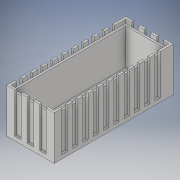
# Autodesk Inventor part: COINTAITER
Saved by Autodesk Inventor 2019 (Build 230136000, 136)
## iProperties
Created: 2020-08-23
Part Number: COINTAITER
Material: Generic
Document SubType Name: Modeling
Designer: mihai
Density: 1 g/cm^3
Appearance: Default
Author: mihai
Autodesk Inventor part; units mm, degrees
ref_plane "YZ Plane" through (0, 0, 0) normal (1, 0, 0) x (0, 1, 0)
ref_plane "XZ Plane" through (0, 0, 0) normal (0, 1, 0) x (-1, 0, 0)
ref_plane "XY Plane" through (0, 0, 0) normal (0, 0, 1) x (1, 0, 0)
sketch "Sketch1" plane through (0, 0, 0) normal (0, 1, 0) x (-1, 0, 0)
  line L0 (0, 0) -> (0, -147.45)
  line L1 (0, -147.45) -> (58.8, -147.45)
  line L2 (58.8, -147.45) -> (58.8, 0)
  line L3 (58.8, 0) -> (0, 0)
  dimension "d0" = 147.45
  dimension "d1" = 58.8
  constraints: 8 end point, 3 perpendicular, 1 vertical
  measures "d0" distance of L0.start L0.end
  measures "d1" distance of L0.end L1.end
extrude "Extrusion1" add sketch "Sketch1" along normal blind 5
sketch "Sketch2" plane through (0, 5, 0) normal (0, 1, 0) x (1, 0, 0)
  line L0 (0, 0) -> (0, 147.45) projected
  line L1 (0, 147.45) -> (-58.8, 147.45) projected
  line L2 (-58.8, 147.45) -> (-58.8, 0) projected
  line L3 (-58.8, 0) -> (0, 0) projected
  line L4 (0, 0) -> (0, 147.45) projected
  line L5 (0, 0) -> (-10, 0)
  line L6 (-10, 0) -> (-10, 5)
  line L7 (-10, 5) -> (-5, 5)
  line L8 (-5, 5) -> (-5, 10)
  line L9 (-5, 10) -> (0, 10)
  line L10 (0, 0) -> (0, 10)
  line L11 (0, 147.45) -> (0, 137.45)
  line L12 (0, 137.45) -> (-5, 137.45)
  line L13 (-5, 137.45) -> (-5, 142.45)
  line L14 (-5, 142.45) -> (-10, 142.45)
  line L15 (-10, 142.45) -> (-10, 147.45)
  line L16 (0, 147.45) -> (-58.8, 147.45) projected
  line L17 (-10, 147.45) -> (0, 147.45)
  line L18 (-58.8, 147.45) -> (-58.8, 137.45)
  line L19 (-53.8, 137.45) -> (-53.8, 142.45)
  line L20 (-53.8, 142.45) -> (-48.8, 142.45)
  line L21 (-48.8, 142.45) -> (-48.8, 147.45)
  line L22 (-48.8, 147.45) -> (-58.8, 147.45)
  line L23 (-58.8, 137.45) -> (-53.8, 137.45)
  line L24 (-58.8, 147.45) -> (-58.8, 0) projected
  line L25 (-58.8, 0) -> (-58.8, 10)
  line L26 (-58.8, 10) -> (-53.8, 10)
  line L27 (-53.8, 10) -> (-53.8, 5)
  line L28 (-53.8, 5) -> (-48.8, 5)
  line L29 (-48.8, 5) -> (-48.8, 0)
  line L30 (-58.8, 0) -> (0, 0) projected
  line L31 (-48.8, 0) -> (-58.8, 0)
  dimension "d7" = 10
  dimension "d8" = 10
  constraints: 48 end point, 13 perpendicular, 10 point on line, 2 collinear, 1 horizontal, 1 parallel, 1 vertical
  measures "d7" distance of L4.start L5.end
  measures "d8" distance of L0.end L11.end
extrude "Extrusion2" add sketch "Sketch2" along normal blind 49.575 contours L3 L6 L7 L8 L9 L0 | L12 L13 L14 L15 L1 L0 | L3 L2 L26 L27 L28 L29 | L21 L20 L19 L23 L2 L1
sketch "Sketch3" plane through (0, 5, 0) normal (0, 1, 0) x (1, 0, 0)
  line L0 (-5, 10) -> (0, 10) projected
  line L1 (-2.5, 10) -> (-2.5, 16.3725) construction
  line L2 (-2.5, 16.3725) -> (-2.5, 22.745) construction
  line L3 (-2.5, 10) -> (-2.5, 16.3725)
  line L4 (-2.5, 16.3725) -> (0, 16.3725)
  line L5 (0, 16.3725) -> (0, 22.745)
  line L6 (0, 22.745) -> (-2.5, 22.745)
  line L7 (-5, 5) -> (-5, 10) projected
  line L8 (-5, 137.45) -> (0, 137.45) projected
  line L9 (-5, 10) -> (-5, 137.45)
  line L10 (-10, 142.45) -> (-10, 147.45) projected
  line L11 (-53.8, 142.45) -> (-48.8, 142.45) projected
  line L12 (-10, 142.45) -> (-48.8, 142.45)
  line L13 (-53.8, 137.45) -> (-53.8, 10)
  line L14 (-48.8, 5) -> (-48.8, 0) projected
  line L15 (-48.8, 5) -> (-10, 5)
  line L16 (-2.5, 22.745) -> (-2.5, 29.1175)
  line L17 (-2.5, 29.1175) -> (0, 29.1175)
  line L18 (0, 29.1175) -> (0, 35.49)
  line L19 (0, 35.49) -> (-2.5, 35.49)
  line L20 (-2.5, 35.49) -> (-2.5, 41.8625)
  line L21 (-2.5, 41.8625) -> (0, 41.8625)
  line L22 (0, 41.8625) -> (0, 48.235)
  line L23 (0, 48.235) -> (-2.5, 48.235)
  line L24 (-2.5, 48.235) -> (-2.5, 54.6075)
  line L25 (-2.5, 54.6075) -> (0, 54.6075)
  line L26 (0, 54.6075) -> (0, 60.98)
  line L27 (0, 60.98) -> (-2.5, 60.98)
  line L28 (-2.5, 60.98) -> (-2.5, 67.3525)
  line L29 (-2.5, 67.3525) -> (0, 67.3525)
  line L30 (0, 67.3525) -> (0, 73.725)
  line L31 (0, 73.725) -> (-2.5, 73.725)
  line L32 (-2.5, 73.725) -> (-2.5, 80.0975)
  line L33 (-2.5, 80.0975) -> (0, 80.0975)
  line L34 (0, 80.0975) -> (0, 86.47)
  line L35 (0, 86.47) -> (-2.5, 86.47)
  line L36 (-2.5, 86.47) -> (-2.5, 92.8425)
  line L37 (-2.5, 92.8425) -> (0, 92.8425)
  line L38 (0, 92.8425) -> (0, 99.215)
  line L39 (0, 99.215) -> (-2.5, 99.215)
  line L40 (-2.5, 99.215) -> (-2.5, 105.5875)
  line L41 (-2.5, 105.5875) -> (0, 105.5875)
  line L42 (0, 105.5875) -> (0, 111.96)
  line L43 (0, 111.96) -> (-2.5, 111.96)
  line L44 (-2.5, 111.96) -> (-2.5, 118.3325)
  line L45 (-2.5, 118.3325) -> (0, 118.3325)
  line L46 (0, 118.3325) -> (0, 124.705)
  line L47 (0, 124.705) -> (-2.5, 124.705)
  line L48 (-2.5, 124.705) -> (-2.5, 131.0775)
  line L49 (-2.5, 131.0775) -> (0, 131.0775)
  line L50 (0, 131.0775) -> (0, 137.45)
  line L51 (0, 137.45) -> (-2.5, 137.45)
  line L52 (-5, 10) -> (-2.5, 10)
  line L53 (0, 10) -> (0, 137.45) projected
  line L54 (-5, 137.45) -> (0, 137.45)
  point P0 (0, 0)
  dimension "d11" = 6.3725
  dimension "d12" = 6.3725
  constraints: 96 end point, 4 horizontal, 4 vertical, 2 collinear, 1 midpoint, 1 perpendicular, 1 other
  measures "d11" distance of L1.start L1.end
  measures "d12" distance of L2.end L1.end
extrude "Extrusion3" add sketch "Sketch3" along normal blind 49.575 contours L9 L8 L50 L49 L48 L47 L46 L45 L44 L43 L42 L41 L40 L39 L38 L37 L36 L35 L34 L33 L32 L31 L30 L29 L28 L27 L26 L25 L24 L23 L22 L21 L20 L19 L18 L17 L16 L6 L5 L4 L3 L0
sketch "Sketch4" plane through (0, 5, 0) normal (0, 1, 0) x (1, 0, 0)
  line L0 (-2.5, 10) -> (-2.5, 16.3725) projected
  line L1 (0, 10) -> (-2.5, 10) projected
  line L2 (-58.8, 10) -> (-53.8, 10) projected
  line L3 (-56.3, 10) -> (-56.3, 16.3725)
  line L4 (-56.3, 16.3725) -> (-58.8, 16.3725)
  line L5 (0, 16.3725) -> (0, 22.745) projected
  line L6 (0, 22.745) -> (-2.5, 22.745) projected
  line L7 (-58.8, 16.3725) -> (-58.8, 22.745)
  line L8 (-58.8, 22.745) -> (-56.3, 22.745)
  line L9 (-5, 142.45) -> (-5, 5) projected
  line L10 (-56.3, 22.745) -> (-56.3, 29.1175)
  line L11 (-56.3, 29.1175) -> (-58.8, 29.1175)
  line L12 (-58.8, 29.1175) -> (-58.8, 35.49)
  line L13 (-58.8, 35.49) -> (-56.3, 35.49)
  line L14 (-56.3, 35.49) -> (-56.3, 41.8625)
  line L15 (-56.3, 41.8625) -> (-58.8, 41.8625)
  line L16 (-58.8, 41.8625) -> (-58.8, 48.235)
  line L17 (-58.8, 48.235) -> (-56.3, 48.235)
  line L18 (-56.3, 48.235) -> (-56.3, 54.6075)
  line L19 (-56.3, 54.6075) -> (-58.8, 54.6075)
  line L20 (-58.8, 54.6075) -> (-58.8, 60.98)
  line L21 (-58.8, 60.98) -> (-56.3, 60.98)
  line L22 (-56.3, 60.98) -> (-56.3, 67.3525)
  line L23 (-56.3, 67.3525) -> (-58.8, 67.3525)
  line L24 (-58.8, 67.3525) -> (-58.8, 73.725)
  line L25 (-58.8, 73.725) -> (-56.3, 73.725)
  line L26 (-56.3, 73.725) -> (-56.3, 80.0975)
  line L27 (-56.3, 80.0975) -> (-58.8, 80.0975)
  line L28 (-58.8, 80.0975) -> (-58.8, 86.47)
  line L29 (-58.8, 86.47) -> (-56.3, 86.47)
  line L30 (-56.3, 86.47) -> (-56.3, 92.8425)
  line L31 (-56.3, 92.8425) -> (-58.8, 92.8425)
  line L32 (-58.8, 92.8425) -> (-58.8, 99.215)
  line L33 (-58.8, 99.215) -> (-56.3, 99.215)
  line L34 (-56.3, 99.215) -> (-56.3, 105.5875)
  line L35 (-56.3, 105.5875) -> (-58.8, 105.5875)
  line L36 (-58.8, 105.5875) -> (-58.8, 111.96)
  line L37 (-58.8, 111.96) -> (-56.3, 111.96)
  line L38 (-56.3, 111.96) -> (-56.3, 118.3325)
  line L39 (-56.3, 118.3325) -> (-58.8, 118.3325)
  line L40 (-58.8, 118.3325) -> (-58.8, 124.705)
  line L41 (-58.8, 124.705) -> (-56.3, 124.705)
  line L42 (-56.3, 124.705) -> (-56.3, 131.0775)
  line L43 (-56.3, 131.0775) -> (-58.8, 131.0775)
  line L44 (-58.8, 131.0775) -> (-58.8, 137.45)
  line L45 (-58.8, 137.45) -> (-56.3, 137.45)
  line L46 (-58.8, 137.45) -> (-53.8, 137.45) projected
  line L47 (-56.3, 137.45) -> (-53.8, 137.45)
  line L48 (-53.8, 137.45) -> (-53.8, 10)
  line L49 (-56.3, 10) -> (-53.8, 10)
  point P0 (0, 0)
  constraints: 86 end point, 2 collinear, 2 perpendicular, 1 horizontal, 1 midpoint, 1 vertical
extrude "Extrusion4" add sketch "Sketch4" along normal blind 49.575
sketch "Sketch5" plane through (0, 5, 0) normal (0, 1, 0) x (1, 0, 0)
  line L0 (-10, 0) -> (-10, 5) projected
  line L1 (-10, 2.5) -> (-17.771, 2.5)
  line L2 (-17.771, 2.5) -> (-17.771, 0)
  line L3 (-17.771, 0) -> (-25.542, 0)
  line L4 (-25.542, 0) -> (-25.542, 2.5)
  line L5 (-5, 5) -> (-10, 5) projected
  line L6 (-25.542, 2.5) -> (-33.313, 2.5)
  line L7 (-33.313, 2.5) -> (-33.313, 0)
  line L8 (-33.313, 0) -> (-41.084, 0)
  line L9 (-48.8, 0) -> (-10, 0) projected
  line L10 (-41.084, 0) -> (-41.084, 2.5)
  line L11 (-41.084, 2.5) -> (-48.8, 2.5)
  line L12 (-48.8, 0) -> (-48.8, 5) projected
  line L13 (-48.8, 2.5) -> (-48.8, 5)
  line L14 (-10, 5) -> (-5, 5) projected
  line L15 (-48.8, 5) -> (-10, 5)
  line L16 (-10, 142.45) -> (-48.8, 142.45)
  line L17 (-48.8, 142.45) -> (-48.8, 144.95)
  line L18 (-41.084, 144.95) -> (-48.8, 144.95)
  line L19 (-41.084, 144.95) -> (-41.084, 147.45)
  line L20 (-41.084, 147.45) -> (-33.313, 147.45)
  line L21 (-33.313, 147.45) -> (-33.313, 144.95)
  line L22 (-33.313, 144.95) -> (-25.542, 144.95)
  line L23 (-25.542, 144.95) -> (-25.542, 147.45)
  line L24 (-25.542, 147.45) -> (-17.771, 147.45)
  line L25 (-17.771, 147.45) -> (-17.771, 144.95)
  line L26 (-17.771, 144.95) -> (-10, 144.95)
  line L27 (-10, 142.45) -> (-10, 147.45) projected
  line L28 (-10, 144.95) -> (-10, 142.45)
  point P0 (0, 0)
  dimension "d31" = 7.771
  dimension "d32" = 7.771
  dimension "d33" = 7.771
  dimension "d34" = 7.771
  constraints: 46 end point, 9 perpendicular, 5 horizontal, 5 point on line, 2 collinear, 2 vertical, 1 midpoint
  measures "d31" distance of L1.start L1.end
  measures "d32" distance of L2.end L3.end
  measures "d33" distance of L4.end L6.end
  measures "d34" distance of L7.end L8.end
extrude "Extrusion5" add sketch "Sketch5" along normal blind 49.575 contours L1 L2 L3 L4 L6 L7 L8 L10 L11 L12 L15 L0 | L16 L17 L18 L19 L20 L21 L22 L23 L24 L25 L26 L27
fillet "Fillet1" radius 1 1 edges at (0, 29.7875, -10)
sketch "Sketch6" plane through (0, 54.575, 0) normal (0, 1, 0) x (1, 0, 0)
  arc A0 (0, 9) -> (-1, 10) centre (-1, 9) ccw projected
  line L0 (-1, 10) -> (-2.5, 10) projected
  line L1 (-2.5, 10) -> (-2.5, 16.3725) projected
  line L2 (-2.5, 16.3725) -> (0, 16.3725) projected
  line L3 (0, 16.3725) -> (0, 22.745) projected
  line L4 (0, 22.745) -> (-2.5, 22.745) projected
  line L5 (-2.5, 22.745) -> (-2.5, 29.1175) projected
  line L6 (-2.5, 29.1175) -> (0, 29.1175) projected
  line L7 (0, 29.1175) -> (0, 35.49) projected
  line L8 (0, 35.49) -> (-2.5, 35.49) projected
  line L9 (-2.5, 35.49) -> (-2.5, 41.8625) projected
  line L10 (-2.5, 41.8625) -> (0, 41.8625) projected
  line L11 (0, 41.8625) -> (0, 48.235) projected
  line L12 (0, 48.235) -> (-2.5, 48.235) projected
  line L13 (-2.5, 48.235) -> (-2.5, 54.6075) projected
  line L14 (-2.5, 54.6075) -> (0, 54.6075) projected
  line L15 (0, 54.6075) -> (0, 60.98) projected
  line L16 (0, 60.98) -> (-2.5, 60.98) projected
  line L17 (-2.5, 60.98) -> (-2.5, 67.3525) projected
  line L18 (-2.5, 67.3525) -> (0, 67.3525) projected
  line L19 (0, 67.3525) -> (0, 73.725) projected
  line L20 (0, 73.725) -> (-2.5, 73.725) projected
  line L21 (-2.5, 73.725) -> (-2.5, 80.0975) projected
  line L22 (-2.5, 80.0975) -> (0, 80.0975) projected
  line L23 (0, 80.0975) -> (0, 86.47) projected
  line L24 (0, 86.47) -> (-2.5, 86.47) projected
  line L25 (-2.5, 86.47) -> (-2.5, 92.8425) projected
  line L26 (-2.5, 92.8425) -> (0, 92.8425) projected
  line L27 (0, 92.8425) -> (0, 99.215) projected
  line L28 (0, 99.215) -> (-2.5, 99.215) projected
  line L29 (-2.5, 99.215) -> (-2.5, 105.5875) projected
  line L30 (-2.5, 105.5875) -> (0, 105.5875) projected
  line L31 (0, 105.5875) -> (0, 111.96) projected
  line L32 (0, 111.96) -> (-2.5, 111.96) projected
  line L33 (-2.5, 111.96) -> (-2.5, 118.3325) projected
  line L34 (-2.5, 118.3325) -> (0, 118.3325) projected
  line L35 (0, 118.3325) -> (0, 124.705) projected
  line L36 (0, 124.705) -> (-2.5, 124.705) projected
  line L37 (-2.5, 124.705) -> (-2.5, 131.0775) projected
  line L38 (-2.5, 131.0775) -> (0, 131.0775) projected
  line L39 (0, 131.0775) -> (0, 147.45) projected
  line L40 (0, 147.45) -> (-10, 147.45) projected
  line L41 (-10, 147.45) -> (-10, 144.95) projected
  line L42 (-10, 144.95) -> (-17.771, 144.95) projected
  line L43 (-17.771, 144.95) -> (-17.771, 147.45) projected
  line L44 (-17.771, 147.45) -> (-25.542, 147.45) projected
  line L45 (-25.542, 147.45) -> (-25.542, 144.95) projected
  line L46 (-25.542, 144.95) -> (-33.313, 144.95) projected
  line L47 (-33.313, 144.95) -> (-33.313, 147.45) projected
  line L48 (-33.313, 147.45) -> (-41.084, 147.45) projected
  line L49 (-41.084, 147.45) -> (-41.084, 144.95) projected
  line L50 (-41.084, 144.95) -> (-48.8, 144.95) projected
  line L51 (-48.8, 144.95) -> (-48.8, 147.45) projected
  line L52 (-48.8, 147.45) -> (-58.8, 147.45) projected
  line L53 (-58.8, 147.45) -> (-58.8, 131.0775) projected
  line L54 (-58.8, 131.0775) -> (-56.3, 131.0775) projected
  line L55 (-56.3, 131.0775) -> (-56.3, 124.705) projected
  line L56 (-56.3, 124.705) -> (-58.8, 124.705) projected
  line L57 (-58.8, 124.705) -> (-58.8, 118.3325) projected
  line L58 (-58.8, 118.3325) -> (-56.3, 118.3325) projected
  line L59 (-56.3, 118.3325) -> (-56.3, 111.96) projected
  line L60 (-56.3, 111.96) -> (-58.8, 111.96) projected
  line L61 (-58.8, 111.96) -> (-58.8, 105.5875) projected
  line L62 (-58.8, 105.5875) -> (-56.3, 105.5875) projected
  line L63 (-56.3, 105.5875) -> (-56.3, 99.215) projected
  line L64 (-56.3, 99.215) -> (-58.8, 99.215) projected
  line L65 (-58.8, 99.215) -> (-58.8, 92.8425) projected
  line L66 (-58.8, 92.8425) -> (-56.3, 92.8425) projected
  line L67 (-56.3, 92.8425) -> (-56.3, 86.47) projected
  line L68 (-56.3, 86.47) -> (-58.8, 86.47) projected
  line L69 (-58.8, 86.47) -> (-58.8, 80.0975) projected
  line L70 (-58.8, 80.0975) -> (-56.3, 80.0975) projected
  line L71 (-56.3, 80.0975) -> (-56.3, 73.725) projected
  line L72 (-56.3, 73.725) -> (-58.8, 73.725) projected
  line L73 (-58.8, 73.725) -> (-58.8, 67.3525) projected
  line L74 (-58.8, 67.3525) -> (-56.3, 67.3525) projected
  line L75 (-56.3, 67.3525) -> (-56.3, 60.98) projected
  line L76 (-56.3, 60.98) -> (-58.8, 60.98) projected
  line L77 (-58.8, 60.98) -> (-58.8, 54.6075) projected
  line L78 (-58.8, 54.6075) -> (-56.3, 54.6075) projected
  line L79 (-56.3, 54.6075) -> (-56.3, 48.235) projected
  line L80 (-56.3, 48.235) -> (-58.8, 48.235) projected
  line L81 (-58.8, 48.235) -> (-58.8, 41.8625) projected
  line L82 (-58.8, 41.8625) -> (-56.3, 41.8625) projected
  line L83 (-56.3, 41.8625) -> (-56.3, 35.49) projected
  line L84 (-56.3, 35.49) -> (-58.8, 35.49) projected
  line L85 (-58.8, 35.49) -> (-58.8, 29.1175) projected
  line L86 (-58.8, 29.1175) -> (-56.3, 29.1175) projected
  line L87 (-56.3, 29.1175) -> (-56.3, 22.745) projected
  line L88 (-56.3, 22.745) -> (-58.8, 22.745) projected
  line L89 (-58.8, 22.745) -> (-58.8, 16.3725) projected
  line L90 (-58.8, 16.3725) -> (-56.3, 16.3725) projected
  line L91 (-56.3, 16.3725) -> (-56.3, 10) projected
  line L92 (-56.3, 10) -> (-58.8, 10) projected
  line L93 (-58.8, 10) -> (-58.8, 0) projected
  line L94 (-58.8, 0) -> (-48.8, 0) projected
  line L95 (-48.8, 0) -> (-48.8, 2.5) projected
  line L96 (-48.8, 2.5) -> (-41.084, 2.5) projected
  line L97 (-41.084, 2.5) -> (-41.084, 0) projected
  line L98 (-41.084, 0) -> (-33.313, 0) projected
  line L99 (-33.313, 0) -> (-33.313, 2.5) projected
  line L100 (-33.313, 2.5) -> (-25.542, 2.5) projected
  line L101 (-25.542, 2.5) -> (-25.542, 0) projected
  line L102 (-25.542, 0) -> (-17.771, 0) projected
  line L103 (-17.771, 0) -> (-17.771, 2.5) projected
  line L104 (-17.771, 2.5) -> (-10, 2.5) projected
  line L105 (-10, 2.5) -> (-10, 0) projected
  line L106 (-10, 0) -> (0, 0) projected
  line L107 (0, 0) -> (0, 9) projected
  line L108 (-5, 5) -> (-53.8, 5) projected
  line L109 (-53.8, 5) -> (-53.8, 142.45) projected
  line L110 (-53.8, 142.45) -> (-5, 142.45) projected
  line L111 (-5, 142.45) -> (-5, 5) projected
  line L112 (-2.5, 144.95) -> (-56.3, 144.95)
  line L113 (-56.3, 144.95) -> (-56.3, 2.5)
  line L114 (-56.3, 2.5) -> (-2.5, 2.5)
  line L115 (-2.5, 2.5) -> (-2.5, 144.95)
  constraints: 8 end point, 2 perpendicular, 1 horizontal, 1 parallel
extrude "Extrusion7" cut sketch "Sketch6" against normal blind 5 contours L115 L114 L104 L100 L96 L113 L91 L87 L83 L79 L75 L71 L67 L63 L59 L55 L112 L50 L46 L42 L37 L33 L29 L25 L21 L17 L13 L9 L5 L1
body "Solid1"
